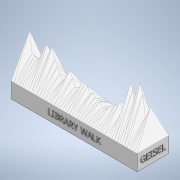
# Autodesk Inventor part: sub_base_fourier
Saved by Autodesk Inventor 2020.1 (Build 241239000, 239)
## iProperties
Created: 2019-10-01
Part Number: sub_base_fourier
Material: Generic
Document SubType Name: Modeling
Designer: Babynado
Density: 1 g/cm^3
Appearance: Default
Author: Babynado
Autodesk Inventor part; units mm, degrees
(part 1 of 3)
ref_plane "YZ Plane" through (0, 0, 0) normal (1, 0, 0) x (0, 1, 0)
ref_plane "XZ Plane" through (0, 0, 0) normal (0, 1, 0) x (-1, 0, 0)
ref_plane "XY Plane" through (0, 0, 0) normal (0, 0, 1) x (1, 0, 0)
sketch "Sketch1" plane through (0, 0, 0) normal (0, 1, 0) x (-1, 0, 0)
  line L0 (0, 0) -> (0, 50.8) projected
  line L1 (0, 50.8) -> (-203.2, 50.8) projected
  line L2 (-203.2, 0) -> (0, 0) projected
  line L3 (-203.2, 50.8) -> (-203.2, 0) projected
extrude "Extrusion1" add sketch "Sketch1" against normal blind 25.4
sketch "Sketch2" plane through (0, 0, 50.8) normal (0, 0, 1) x (1, 0, 0)
  line L0 (0, 0) -> (203.2, 0) projected
  line L1 (0, 0) -> (203.2, 0) projected
  line L2 (0, 0) -> (0, -25.4) projected
  line L3 (203.2, -25.4) -> (0, -25.4) projected
  line L4 (203.2, 0) -> (203.2, -25.4) projected
  line L5 (50.8, -8.636) -> (152.4, -8.636) construction
  line L6 (152.4, -8.636) -> (152.4, -16.764) construction
  line L7 (152.4, -16.764) -> (50.8, -16.764) construction
  line L8 (50.8, -16.764) -> (50.8, -8.636) construction
  line L9 (65.2204, -17.272) -> (59.9222, -17.272)
  line L10 (59.9222, -17.272) -> (59.9222, -8.128)
  line L11 (59.9222, -8.128) -> (61.1374, -8.128)
  line L12 (61.1374, -8.128) -> (61.1374, -16.1901)
  line L13 (61.1374, -16.1901) -> (65.2204, -16.1901)
  line L14 (65.2204, -16.1901) -> (65.2204, -17.272)
  line L15 (69.3626, -17.272) -> (65.8206, -17.272)
  line L16 (65.8206, -17.272) -> (65.8206, -16.3383)
  line L17 (65.8206, -16.3383) -> (66.984, -16.3383)
  line L18 (66.984, -16.3383) -> (66.984, -9.0617)
  line L19 (66.984, -9.0617) -> (65.8206, -9.0617)
  line L20 (65.8206, -9.0617) -> (65.8206, -8.128)
  line L21 (65.8206, -8.128) -> (69.3626, -8.128)
  line L22 (69.3626, -8.128) -> (69.3626, -9.0617)
  line L23 (69.3626, -9.0617) -> (68.1992, -9.0617)
  line L24 (68.1992, -9.0617) -> (68.1992, -16.3383)
  line L25 (68.1992, -16.3383) -> (69.3626, -16.3383)
  line L26 (69.3626, -16.3383) -> (69.3626, -17.272)
  spline S0 degree 2 poles (77.069, -14.4636) (77.069, -15.1453) (76.5503, -16.1901) (76.1205, -16.531) knots 0 0 0 1 2 2 2
  spline S1 degree 2 poles (76.1205, -16.531) (75.6018, -16.9311) (74.4236, -17.272) (73.49, -17.272) knots 0 0 0 1 2 2 2
  line L27 (73.49, -17.272) -> (70.8668, -17.272)
  line L28 (70.8668, -17.272) -> (70.8668, -8.128)
  line L29 (70.8668, -8.128) -> (73.2899, -8.128)
  spline S2 degree 2 poles (73.2899, -8.128) (74.268, -8.128) (75.2462, -8.254) (75.6908, -8.4985) knots 0 0 0 1 2 2 2
  spline S3 degree 2 poles (75.6908, -8.4985) (76.1872, -8.7579) (76.6392, -9.61) (76.6392, -10.188) knots 0 0 0 1 2 2 2
  spline S4 degree 2 poles (76.6392, -10.188) (76.6392, -10.8327) (75.9575, -11.8553) (75.3573, -12.1442) knots 0 0 0 1 2 2 2
  line L30 (75.3573, -12.1442) -> (75.3573, -12.1887)
  spline S5 degree 2 poles (75.3573, -12.1887) (76.1724, -12.411) (77.069, -13.5892) (77.069, -14.4636) knots 0 0 0 1 2 2 2
  spline S6 degree 2 poles (75.8019, -14.5155) (75.8019, -13.9968) (75.5055, -13.3299) (75.0609, -13.0927) knots 0 0 0 1 2 2 2
  spline S7 degree 2 poles (75.0609, -13.0927) (74.7719, -12.9445) (74.0902, -12.8556) (73.4603, -12.8556) knots 0 0 0 1 2 2 2
  line L31 (73.4603, -12.8556) -> (72.0821, -12.8556)
  line L32 (72.0821, -12.8556) -> (72.0821, -16.2346)
  line L33 (72.0821, -16.2346) -> (73.0676, -16.2346)
  spline S8 degree 2 poles (73.0676, -16.2346) (73.8679, -16.2346) (74.7867, -16.0864) (75.1424, -15.8493) knots 0 0 0 1 2 2 2
  spline S9 degree 2 poles (75.1424, -15.8493) (75.4833, -15.6047) (75.8019, -14.9971) (75.8019, -14.5155) knots 0 0 0 1 2 2 2
  spline S10 degree 2 poles (75.3721, -10.3584) (75.3721, -10.0324) (75.1498, -9.5433) (74.9053, -9.4025) knots 0 0 0 1 2 2 2
  spline S11 degree 2 poles (74.9053, -9.4025) (74.6089, -9.2395) (73.8901, -9.1654) (73.2454, -9.1654) knots 0 0 0 1 2 2 2
  line L34 (73.2454, -9.1654) -> (72.0821, -9.1654)
  line L35 (72.0821, -9.1654) -> (72.0821, -11.8404)
  line L36 (72.0821, -11.8404) -> (73.4603, -11.8404)
  spline S12 degree 2 poles (73.4603, -11.8404) (74.0309, -11.8404) (74.5718, -11.7219) (74.8608, -11.5366) knots 0 0 0 1 2 2 2
  spline S13 degree 2 poles (74.8608, -11.5366) (75.1424, -11.3588) (75.3721, -10.7882) (75.3721, -10.3584) knots 0 0 0 1 2 2 2
  line L37 (85.3535, -17.272) -> (83.7751, -17.272)
  line L38 (83.7751, -17.272) -> (80.8852, -13.6337)
  line L39 (80.8852, -13.6337) -> (79.4921, -13.6337)
  line L40 (79.4921, -13.6337) -> (79.4921, -17.272)
  line L41 (79.4921, -17.272) -> (78.2769, -17.272)
  line L42 (78.2769, -17.272) -> (78.2769, -8.128)
  line L43 (78.2769, -8.128) -> (80.6333, -8.128)
  spline S14 degree 2 poles (80.6333, -8.128) (81.4187, -8.128) (82.4784, -8.2984) (82.96, -8.6097) knots 0 0 0 1 2 2 2
  spline S15 degree 2 poles (82.96, -8.6097) (83.4417, -8.9209) (83.9974, -9.8916) (83.9974, -10.6104) knots 0 0 0 1 2 2 2
  spline S16 degree 2 poles (83.9974, -10.6104) (83.9974, -11.6107) (82.9748, -12.9668) (82.1005, -13.2928) knots 0 0 0 1 2 2 2
  line L44 (82.1005, -13.2928) -> (85.3535, -17.272)
  spline S17 degree 2 poles (82.7303, -10.7067) (82.7303, -10.3066) (82.4487, -9.6915) (82.1523, -9.4914) knots 0 0 0 1 2 2 2
  spline S18 degree 2 poles (82.1523, -9.4914) (81.893, -9.321) (81.2038, -9.1802) (80.7, -9.1802) knots 0 0 0 1 2 2 2
  line L45 (80.7, -9.1802) -> (79.4921, -9.1802)
  line L46 (79.4921, -9.1802) -> (79.4921, -12.6185)
  line L47 (79.4921, -12.6185) -> (80.5592, -12.6185)
  spline S19 degree 2 poles (80.5592, -12.6185) (81.0853, -12.6185) (81.9226, -12.4332) (82.2116, -12.1442) knots 0 0 0 1 2 2 2
  spline S20 degree 2 poles (82.2116, -12.1442) (82.4784, -11.8923) (82.7303, -11.1809) (82.7303, -10.7067) knots 0 0 0 1 2 2 2
  line L48 (85.0941, -17.272) -> (88.1767, -8.128)
  line L49 (88.1767, -8.128) -> (89.6735, -8.128)
  line L50 (89.6735, -8.128) -> (92.7561, -17.272)
  line L51 (92.7561, -17.272) -> (91.4742, -17.272)
  line L52 (91.4742, -17.272) -> (90.6442, -14.7155)
  line L53 (90.6442, -14.7155) -> (87.1541, -14.7155)
  line L54 (87.1541, -14.7155) -> (86.3242, -17.272)
  line L55 (86.3242, -17.272) -> (85.0941, -17.272)
  line L56 (90.3108, -13.6781) -> (88.8955, -9.3729)
  line L57 (88.8955, -9.3729) -> (87.4876, -13.6781)
  line L58 (87.4876, -13.6781) -> (90.3108, -13.6781)
  line L59 (100.6997, -17.272) -> (99.1213, -17.272)
  line L60 (99.1213, -17.272) -> (96.2314, -13.6337)
  line L61 (96.2314, -13.6337) -> (94.8383, -13.6337)
  line L62 (94.8383, -13.6337) -> (94.8383, -17.272)
  line L63 (94.8383, -17.272) -> (93.6231, -17.272)
  line L64 (93.6231, -17.272) -> (93.6231, -8.128)
  line L65 (93.6231, -8.128) -> (95.9795, -8.128)
  spline S21 degree 2 poles (95.9795, -8.128) (96.7649, -8.128) (97.8246, -8.2984) (98.3062, -8.6097) knots 0 0 0 1 2 2 2
  spline S22 degree 2 poles (98.3062, -8.6097) (98.7879, -8.9209) (99.3436, -9.8916) (99.3436, -10.6104) knots 0 0 0 1 2 2 2
  spline S23 degree 2 poles (99.3436, -10.6104) (99.3436, -11.6107) (98.3211, -12.9668) (97.4467, -13.2928) knots 0 0 0 1 2 2 2
  line L66 (97.4467, -13.2928) -> (100.6997, -17.272)
  spline S24 degree 2 poles (98.0765, -10.7067) (98.0765, -10.3066) (97.7949, -9.6915) (97.4985, -9.4914) knots 0 0 0 1 2 2 2
  spline S25 degree 2 poles (97.4985, -9.4914) (97.2392, -9.321) (96.55, -9.1802) (96.0462, -9.1802) knots 0 0 0 1 2 2 2
  line L67 (96.0462, -9.1802) -> (94.8383, -9.1802)
  line L68 (94.8383, -9.1802) -> (94.8383, -12.6185)
  line L69 (94.8383, -12.6185) -> (95.9054, -12.6185)
  spline S26 degree 2 poles (95.9054, -12.6185) (96.4315, -12.6185) (97.2688, -12.4332) (97.5578, -12.1442) knots 0 0 0 1 2 2 2
  spline S27 degree 2 poles (97.5578, -12.1442) (97.8246, -11.8923) (98.0765, -11.1809) (98.0765, -10.7067) knots 0 0 0 1 2 2 2
  line L70 (107.8281, -8.128) -> (104.7382, -13.2261)
  line L71 (104.7382, -13.2261) -> (104.7382, -17.272)
  line L72 (104.7382, -17.272) -> (103.5229, -17.272)
  line L73 (103.5229, -17.272) -> (103.5229, -13.3521)
  line L74 (103.5229, -13.3521) -> (100.4329, -8.128)
  line L75 (100.4329, -8.128) -> (101.7815, -8.128)
  line L76 (101.7815, -8.128) -> (104.1379, -12.1517)
  line L77 (104.1379, -12.1517) -> (106.5388, -8.128)
  line L78 (106.5388, -8.128) -> (107.8281, -8.128)
  line L79 (122.8483, -8.128) -> (120.5512, -17.272)
  line L80 (120.5512, -17.272) -> (119.1877, -17.272)
  line L81 (119.1877, -17.272) -> (117.3278, -9.6841)
  line L82 (117.3278, -9.6841) -> (115.5198, -17.272)
  line L83 (115.5198, -17.272) -> (114.1711, -17.272)
  line L84 (114.1711, -17.272) -> (111.837, -8.128)
  line L85 (111.837, -8.128) -> (113.0893, -8.128)
  line L86 (113.0893, -8.128) -> (114.927, -15.7085)
  line L87 (114.927, -15.7085) -> (116.7498, -8.128)
  line L88 (116.7498, -8.128) -> (117.9873, -8.128)
  line L89 (117.9873, -8.128) -> (119.825, -15.7974)
  line L90 (119.825, -15.7974) -> (121.6553, -8.128)
  line L91 (121.6553, -8.128) -> (122.8483, -8.128)
  line L92 (122.9521, -17.272) -> (126.0346, -8.128)
  line L93 (126.0346, -8.128) -> (127.5315, -8.128)
  line L94 (127.5315, -8.128) -> (130.614, -17.272)
  line L95 (130.614, -17.272) -> (129.3321, -17.272)
  line L96 (129.3321, -17.272) -> (128.5022, -14.7155)
  line L97 (128.5022, -14.7155) -> (125.012, -14.7155)
  line L98 (125.012, -14.7155) -> (124.1821, -17.272)
  line L99 (124.1821, -17.272) -> (122.9521, -17.272)
  line L100 (128.1687, -13.6781) -> (126.7534, -9.3729)
  line L101 (126.7534, -9.3729) -> (125.3455, -13.6781)
  line L102 (125.3455, -13.6781) -> (128.1687, -13.6781)
  line L103 (136.7792, -17.272) -> (131.481, -17.272)
  line L104 (131.481, -17.272) -> (131.481, -8.128)
  line L105 (131.481, -8.128) -> (132.6963, -8.128)
  line L106 (132.6963, -8.128) -> (132.6963, -16.1901)
  line L107 (132.6963, -16.1901) -> (136.7792, -16.1901)
  line L108 (136.7792, -16.1901) -> (136.7792, -17.272)
  line L109 (144.4041, -17.272) -> (142.8258, -17.272)
  line L110 (142.8258, -17.272) -> (139.4839, -13.0186)
  line L111 (139.4839, -13.0186) -> (138.9503, -13.6188)
  line L112 (138.9503, -13.6188) -> (138.9503, -17.272)
  line L113 (138.9503, -17.272) -> (137.7351, -17.272)
  line L114 (137.7351, -17.272) -> (137.7351, -8.128)
  line L115 (137.7351, -8.128) -> (138.9503, -8.128)
  line L116 (138.9503, -8.128) -> (138.9503, -12.3295)
  line L117 (138.9503, -12.3295) -> (142.6998, -8.128)
  line L118 (142.6998, -8.128) -> (144.1818, -8.128)
  line L119 (144.1818, -8.128) -> (140.3953, -12.2109)
  line L120 (140.3953, -12.2109) -> (144.4041, -17.272)
  dimension "d31" = 76.2
  dimension "d2" = 203.2
  dimension "d3" = 25.4
  dimension "d4" = 101.6
  dimension "d5" = 8.128
  dimension "d6" = 8.636
  dimension "d7" = 50.8
  constraints: 2 other
  measures "d2" distance of L0.start L0.end
  measures "d3" distance of L1.start L2.end
  measures "d4" distance of L5.start L5.end
  measures "d5" distance of L7.end L5.start
  measures "d6" distance between parallel lines of L0 L5
  measures "d7" distance between parallel lines of L2 L8
extrude "Extrusion2" cut sketch "Sketch2" against normal blind 5.08 contours L9 L10 L11 L12 L13 L14 | L15 L16 L17 L18 L19 L20 L21 L22 L23 L24 L25 L26 | S0 S1 L27 L28 L29 S2 S3 S4 L30 S5 | L37 L48 L44 | L44 L48 L49 L50 L51 L52 L53 L54 L55 | L37 L38 L39 L40 L41 L42 L43 S14 S15 S16 L44 L48 | L59 L60 L61 L62 L63 L64 L65 S21 S22 S23 L66 | L70 L71 L72 L73 L74 L75 L76 L77 L78 | L79 L80 L81 L82 L83 L84 L85 L86 L87 L88 L89 L90 L91 | L92 L93 L94 L95 L96 L97 L98 L99 | L103 L104 L105 L106 L107 L108 | L109 L110 L111 L112 L113 L114 L115 L116 L117 L118 L119 L120
sketch "Sketch3" plane through (203.2, 0, 50.8) normal (1, 0, 0) x (0, 0, -1)
  line L0 (0, 0) -> (50.8, 0) projected
  line L1 (0, 0) -> (0, -25.4) projected
  line L2 (50.8, -25.4) -> (0, -25.4) projected
  line L3 (50.8, 0) -> (50.8, -25.4) projected
  line L4 (6.35, -5.08) -> (44.45, -5.08) construction
  line L5 (44.45, -5.08) -> (44.45, -20.32) construction
  line L6 (44.45, -20.32) -> (6.35, -20.32) construction
  line L7 (6.35, -20.32) -> (6.35, -5.08) construction
  spline S0 degree 2 poles (9.9315, -17.4424) (8.9608, -17.4424) (7.3528, -16.8496) (6.7748, -16.2494) knots 0 0 0 1 2 2 2
  spline S1 degree 2 poles (6.7748, -16.2494) (6.1969, -15.6418) (5.5818, -13.8486) (5.5818, -12.6852) knots 0 0 0 1 2 2 2
  spline S2 degree 2 poles (5.5818, -12.6852) (5.5818, -11.5811) (6.2043, -9.8323) (6.7823, -9.2099) knots 0 0 0 1 2 2 2
  spline S3 degree 2 poles (6.7823, -9.2099) (7.338, -8.6097) (8.9682, -7.9576) (9.9389, -7.9576) knots 0 0 0 1 2 2 2
  spline S4 degree 2 poles (9.9389, -7.9576) (10.4058, -7.9576) (11.2505, -8.0909) (11.6358, -8.2095) knots 0 0 0 1 2 2 2
  spline S5 degree 2 poles (11.6358, -8.2095) (11.9471, -8.2984) (12.7029, -8.6245) (12.9326, -8.743) knots 0 0 0 1 2 2 2
  line L8 (12.9326, -8.743) -> (12.9326, -10.2102)
  line L9 (12.9326, -10.2102) -> (12.8289, -10.2102)
  spline S6 degree 2 poles (12.8289, -10.2102) (12.5991, -10.0102) (12.1175, -9.6471) (11.6729, -9.4396) knots 0 0 0 1 2 2 2
  spline S7 degree 2 poles (11.6729, -9.4396) (11.3024, -9.2543) (10.3465, -9.0098) (9.7981, -9.0098) knots 0 0 0 1 2 2 2
  spline S8 degree 2 poles (9.7981, -9.0098) (8.4792, -9.0098) (6.8489, -10.9957) (6.8489, -12.6481) knots 0 0 0 1 2 2 2
  spline S9 degree 2 poles (6.8489, -12.6481) (6.8489, -13.567) (7.2787, -14.9452) (7.6863, -15.4195) knots 0 0 0 1 2 2 2
  spline S10 degree 2 poles (7.6863, -15.4195) (8.079, -15.8937) (9.1905, -16.3902) (9.8871, -16.3902) knots 0 0 0 1 2 2 2
  spline S11 degree 2 poles (9.8871, -16.3902) (10.3984, -16.3902) (11.4209, -16.242) (11.7692, -16.0938) knots 0 0 0 1 2 2 2
  line L10 (11.7692, -16.0938) -> (11.7692, -13.73)
  line L11 (11.7692, -13.73) -> (9.6499, -13.73)
  line L12 (9.6499, -13.73) -> (9.6499, -12.6629)
  line L13 (9.6499, -12.6629) -> (12.9696, -12.6629)
  line L14 (12.9696, -12.6629) -> (12.9696, -16.657)
  spline S12 degree 2 poles (12.9696, -16.657) (12.7399, -16.7607) (11.9545, -17.0793) (11.621, -17.1757) knots 0 0 0 1 2 2 2
  spline S13 degree 2 poles (11.621, -17.1757) (11.169, -17.3091) (10.4428, -17.4424) (9.9315, -17.4424) knots 0 0 0 1 2 2 2
  line L15 (14.4961, -17.2646) -> (14.4961, -8.1206)
  line L16 (14.4961, -8.1206) -> (20.2167, -8.1206)
  line L17 (20.2167, -8.1206) -> (20.2167, -9.2025)
  line L18 (20.2167, -9.2025) -> (15.7114, -9.2025)
  line L19 (15.7114, -9.2025) -> (15.7114, -11.7071)
  line L20 (15.7114, -11.7071) -> (19.9129, -11.7071)
  line L21 (19.9129, -11.7071) -> (19.9129, -12.7889)
  line L22 (19.9129, -12.7889) -> (15.7114, -12.7889)
  line L23 (15.7114, -12.7889) -> (15.7114, -16.1827)
  line L24 (15.7114, -16.1827) -> (20.2167, -16.1827)
  line L25 (20.2167, -16.1827) -> (20.2167, -17.2646)
  line L26 (20.2167, -17.2646) -> (14.4961, -17.2646)
  line L27 (24.7368, -17.2646) -> (21.1948, -17.2646)
  line L28 (21.1948, -17.2646) -> (21.1948, -16.3309)
  line L29 (21.1948, -16.3309) -> (22.3582, -16.3309)
  line L30 (22.3582, -16.3309) -> (22.3582, -9.0543)
  line L31 (22.3582, -9.0543) -> (21.1948, -9.0543)
  line L32 (21.1948, -9.0543) -> (21.1948, -8.1206)
  line L33 (21.1948, -8.1206) -> (24.7368, -8.1206)
  line L34 (24.7368, -8.1206) -> (24.7368, -9.0543)
  line L35 (24.7368, -9.0543) -> (23.5734, -9.0543)
  line L36 (23.5734, -9.0543) -> (23.5734, -16.3309)
  line L37 (23.5734, -16.3309) -> (24.7368, -16.3309)
  line L38 (24.7368, -16.3309) -> (24.7368, -17.2646)
  spline S14 degree 2 poles (28.7901, -17.4276) (27.7972, -17.4276) (26.4041, -17.0126) (25.789, -16.7162) knots 0 0 0 1 2 2 2
  line L39 (25.789, -16.7162) -> (25.789, -15.1898)
  line L40 (25.789, -15.1898) -> (25.8779, -15.1898)
  spline S15 degree 2 poles (25.8779, -15.1898) (26.4782, -15.7529) (27.9972, -16.3754) (28.7012, -16.3754) knots 0 0 0 1 2 2 2
  spline S16 degree 2 poles (28.7012, -16.3754) (29.7089, -16.3754) (30.7389, -15.538) (30.7389, -14.8489) knots 0 0 0 1 2 2 2
  spline S17 degree 2 poles (30.7389, -14.8489) (30.7389, -14.3006) (30.198, -13.6188) (29.6126, -13.4484) knots 0 0 0 1 2 2 2
  spline S18 degree 2 poles (29.6126, -13.4484) (29.1902, -13.3299) (28.4863, -13.1668) (27.9602, -13.0335) knots 0 0 0 1 2 2 2
  spline S19 degree 2 poles (27.9602, -13.0335) (27.4859, -12.9075) (26.7375, -12.5296) (26.4485, -12.2258) knots 0 0 0 1 2 2 2
  spline S20 degree 2 poles (26.4485, -12.2258) (26.1669, -11.9219) (25.8557, -11.1068) (25.8557, -10.5733) knots 0 0 0 1 2 2 2
  spline S21 degree 2 poles (25.8557, -10.5733) (25.8557, -9.4618) (27.5897, -7.9576) (28.9309, -7.9576) knots 0 0 0 1 2 2 2
  spline S22 degree 2 poles (28.9309, -7.9576) (29.7015, -7.9576) (31.065, -8.2614) (31.6504, -8.5504) knots 0 0 0 1 2 2 2
  line L41 (31.6504, -8.5504) -> (31.6504, -10.0027)
  line L42 (31.6504, -10.0027) -> (31.5615, -10.0027)
  spline S23 degree 2 poles (31.5615, -10.0027) (31.1243, -9.6026) (29.7608, -9.0098) (29.0124, -9.0098) knots 0 0 0 1 2 2 2
  spline S24 degree 2 poles (29.0124, -9.0098) (28.1677, -9.0098) (27.1228, -9.8027) (27.1228, -10.4473) knots 0 0 0 1 2 2 2
  spline S25 degree 2 poles (27.1228, -10.4473) (27.1228, -11.0253) (27.7379, -11.7145) (28.3159, -11.8701) knots 0 0 0 1 2 2 2
  spline S26 degree 2 poles (28.3159, -11.8701) (28.7012, -11.9738) (29.8201, -12.2406) (30.1906, -12.3517) knots 0 0 0 1 2 2 2
  spline S27 degree 2 poles (30.1906, -12.3517) (31.1317, -12.6407) (32.0061, -13.8041) (32.0061, -14.6563) knots 0 0 0 1 2 2 2
  spline S28 degree 2 poles (32.0061, -14.6563) (32.0061, -15.1972) (31.5689, -16.2346) (31.1761, -16.5977) knots 0 0 0 1 2 2 2
  spline S29 degree 2 poles (31.1761, -16.5977) (30.7389, -16.9978) (29.6274, -17.4276) (28.7901, -17.4276) knots 0 0 0 1 2 2 2
  line L43 (33.2435, -17.2646) -> (33.2435, -8.1206)
  line L44 (33.2435, -8.1206) -> (38.9641, -8.1206)
  line L45 (38.9641, -8.1206) -> (38.9641, -9.2025)
  line L46 (38.9641, -9.2025) -> (34.4588, -9.2025)
  line L47 (34.4588, -9.2025) -> (34.4588, -11.7071)
  line L48 (34.4588, -11.7071) -> (38.6603, -11.7071)
  line L49 (38.6603, -11.7071) -> (38.6603, -12.7889)
  line L50 (38.6603, -12.7889) -> (34.4588, -12.7889)
  line L51 (34.4588, -12.7889) -> (34.4588, -16.1827)
  line L52 (34.4588, -16.1827) -> (38.9641, -16.1827)
  line L53 (38.9641, -16.1827) -> (38.9641, -17.2646)
  line L54 (38.9641, -17.2646) -> (33.2435, -17.2646)
  line L55 (45.5961, -17.2646) -> (40.2979, -17.2646)
  line L56 (40.2979, -17.2646) -> (40.2979, -8.1206)
  line L57 (40.2979, -8.1206) -> (41.5131, -8.1206)
  line L58 (41.5131, -8.1206) -> (41.5131, -16.1827)
  line L59 (41.5131, -16.1827) -> (45.5961, -16.1827)
  line L60 (45.5961, -16.1827) -> (45.5961, -17.2646)
  dimension "d10" = 50.8
  dimension "d11" = 25.4
  dimension "d12" = 38.1
  dimension "d13" = 15.24
  dimension "d14" = 6.35
  dimension "d15" = 5.08
  constraints: 2 other
  measures "d10" distance of L0.start L0.end
  measures "d11" distance of L0.start L1.end
  measures "d12" distance of L4.start L4.end
  measures "d13" distance of L6.end L4.start
  measures "d14" distance between parallel lines of L1 L7
  measures "d15" distance between parallel lines of L2 L6
extrude "Extrusion3" cut sketch "Sketch3" against normal blind 5.08 contours S0 S1 S2 S3 S4 S5 L8 L9 S6 S7 S8 S9 S10 S11 L10 L11 L12 L13 L14 S12 S13 | L15 L16 L17 L18 L19 L20 L21 L22 L23 L24 L25 L26 | L27 L28 L29 L30 L31 L32 L33 L34 L35 L36 L37 L38 | S14 L39 L40 S15 S16 S17 S18 S19 S20 S21 S22 L41 L42 S23 S24 S25 S26 S27 S28 S29 | L43 L44 L45 L46 L47 L48 L49 L50 L51 L52 L53 L54 | L55 L56 L57 L58 L59 L60
sketch "Sketch4" plane through (203.2, 0, 0) normal (0, 0, -1) x (-1, 0, 0)
  line L0 (0, 0) -> (203.2, 0) projected
  line L1 (0, 0) -> (0, -25.4) projected
  line L2 (203.2, -25.4) -> (0, -25.4) projected
  line L3 (203.2, 0) -> (203.2, -25.4) projected
  line L4 (0, -7.62) -> (203.2, -7.62) construction
  line L5 (203.2, -7.62) -> (203.2, -17.78) construction
  line L6 (203.2, -17.78) -> (0, -17.78) construction
  line L7 (0, -17.78) -> (0, -7.62) construction
  spline S0 degree 2 poles (11.9829, -17.435) (10.9899, -17.435) (9.5968, -17.0201) (8.9818, -16.7237) knots 0 0 0 1 2 2 2
  line L8 (8.9818, -16.7237) -> (8.9818, -15.1972)
  line L9 (8.9818, -15.1972) -> (9.0707, -15.1972)
  spline S1 degree 2 poles (9.0707, -15.1972) (9.6709, -15.7604) (11.19, -16.3828) (11.894, -16.3828) knots 0 0 0 1 2 2 2
  spline S2 degree 2 poles (11.894, -16.3828) (12.9017, -16.3828) (13.9317, -15.5455) (13.9317, -14.8563) knots 0 0 0 1 2 2 2
  spline S3 degree 2 poles (13.9317, -14.8563) (13.9317, -14.308) (13.3908, -13.6263) (12.8054, -13.4558) knots 0 0 0 1 2 2 2
  spline S4 degree 2 poles (12.8054, -13.4558) (12.383, -13.3373) (11.6791, -13.1742) (11.153, -13.0409) knots 0 0 0 1 2 2 2
  spline S5 degree 2 poles (11.153, -13.0409) (10.6787, -12.9149) (9.9303, -12.537) (9.6413, -12.2332) knots 0 0 0 1 2 2 2
  spline S6 degree 2 poles (9.6413, -12.2332) (9.3597, -11.9294) (9.0485, -11.1142) (9.0485, -10.5807) knots 0 0 0 1 2 2 2
  spline S7 degree 2 poles (9.0485, -10.5807) (9.0485, -9.4692) (10.7825, -7.965) (12.1237, -7.965) knots 0 0 0 1 2 2 2
  spline S8 degree 2 poles (12.1237, -7.965) (12.8943, -7.965) (14.2578, -8.2688) (14.8432, -8.5578) knots 0 0 0 1 2 2 2
  line L10 (14.8432, -8.5578) -> (14.8432, -10.0102)
  line L11 (14.8432, -10.0102) -> (14.7542, -10.0102)
  spline S9 degree 2 poles (14.7542, -10.0102) (14.317, -9.61) (12.9536, -9.0172) (12.2052, -9.0172) knots 0 0 0 1 2 2 2
  spline S10 degree 2 poles (12.2052, -9.0172) (11.3604, -9.0172) (10.3156, -9.8101) (10.3156, -10.4548) knots 0 0 0 1 2 2 2
  spline S11 degree 2 poles (10.3156, -10.4548) (10.3156, -11.0327) (10.9307, -11.7219) (11.5086, -11.8775) knots 0 0 0 1 2 2 2
  spline S12 degree 2 poles (11.5086, -11.8775) (11.894, -11.9812) (13.0129, -12.248) (13.3834, -12.3591) knots 0 0 0 1 2 2 2
  spline S13 degree 2 poles (13.3834, -12.3591) (14.3245, -12.6481) (15.1988, -13.8115) (15.1988, -14.6637) knots 0 0 0 1 2 2 2
  spline S14 degree 2 poles (15.1988, -14.6637) (15.1988, -15.2046) (14.7616, -16.242) (14.3689, -16.6051) knots 0 0 0 1 2 2 2
  spline S15 degree 2 poles (14.3689, -16.6051) (13.9317, -17.0052) (12.8202, -17.435) (11.9829, -17.435) knots 0 0 0 1 2 2 2
  spline S16 degree 2 poles (19.6301, -17.4647) (18.8224, -17.4647) (17.6219, -17.0423) (17.1996, -16.6199) knots 0 0 0 1 2 2 2
  spline S17 degree 2 poles (17.1996, -16.6199) (16.7179, -16.1457) (16.3252, -14.8119) (16.3252, -13.8337) knots 0 0 0 1 2 2 2
  line L12 (16.3252, -13.8337) -> (16.3252, -8.128)
  line L13 (16.3252, -8.128) -> (17.5404, -8.128)
  line L14 (17.5404, -8.128) -> (17.5404, -13.8337)
  spline S18 degree 2 poles (17.5404, -13.8337) (17.5404, -14.471) (17.7034, -15.3306) (17.9331, -15.6788) knots 0 0 0 1 2 2 2
  spline S19 degree 2 poles (17.9331, -15.6788) (18.1777, -16.0493) (19.0224, -16.4273) (19.6301, -16.4273) knots 0 0 0 1 2 2 2
  spline S20 degree 2 poles (19.6301, -16.4273) (20.2006, -16.4273) (21.0898, -16.0493) (21.3344, -15.6788) knots 0 0 0 1 2 2 2
  spline S21 degree 2 poles (21.3344, -15.6788) (21.5641, -15.3306) (21.7271, -14.4784) (21.7271, -13.8634) knots 0 0 0 1 2 2 2
  line L15 (21.7271, -13.8634) -> (21.7271, -8.128)
  line L16 (21.7271, -8.128) -> (22.9423, -8.128)
  line L17 (22.9423, -8.128) -> (22.9423, -13.8337)
  spline S22 degree 2 poles (22.9423, -13.8337) (22.9423, -14.7896) (22.557, -16.1531) (22.068, -16.6199) knots 0 0 0 1 2 2 2
  spline S23 degree 2 poles (22.068, -16.6199) (21.6308, -17.0497) (20.4748, -17.4647) (19.6301, -17.4647) knots 0 0 0 1 2 2 2
  spline S24 degree 2 poles (30.8859, -14.4636) (30.8859, -15.1453) (30.3672, -16.1901) (29.9374, -16.531) knots 0 0 0 1 2 2 2
  spline S25 degree 2 poles (29.9374, -16.531) (29.4187, -16.9311) (28.2405, -17.272) (27.3069, -17.272) knots 0 0 0 1 2 2 2
  line L18 (27.3069, -17.272) -> (24.6837, -17.272)
  line L19 (24.6837, -17.272) -> (24.6837, -8.128)
  line L20 (24.6837, -8.128) -> (27.1068, -8.128)
  spline S26 degree 2 poles (27.1068, -8.128) (28.0849, -8.128) (29.063, -8.254) (29.5076, -8.4985) knots 0 0 0 1 2 2 2
  spline S27 degree 2 poles (29.5076, -8.4985) (30.0041, -8.7579) (30.4561, -9.61) (30.4561, -10.188) knots 0 0 0 1 2 2 2
  spline S28 degree 2 poles (30.4561, -10.188) (30.4561, -10.8327) (29.7744, -11.8553) (29.1742, -12.1442) knots 0 0 0 1 2 2 2
  line L21 (29.1742, -12.1442) -> (29.1742, -12.1887)
  spline S29 degree 2 poles (29.1742, -12.1887) (29.9893, -12.411) (30.8859, -13.5892) (30.8859, -14.4636) knots 0 0 0 1 2 2 2
  spline S30 degree 2 poles (29.6188, -14.5155) (29.6188, -13.9968) (29.3224, -13.3299) (28.8778, -13.0927) knots 0 0 0 1 2 2 2
  spline S31 degree 2 poles (28.8778, -13.0927) (28.5888, -12.9445) (27.9071, -12.8556) (27.2772, -12.8556) knots 0 0 0 1 2 2 2
  line L22 (27.2772, -12.8556) -> (25.899, -12.8556)
  line L23 (25.899, -12.8556) -> (25.899, -16.2346)
  line L24 (25.899, -16.2346) -> (26.8845, -16.2346)
  spline S32 degree 2 poles (26.8845, -16.2346) (27.6848, -16.2346) (28.6036, -16.0864) (28.9593, -15.8493) knots 0 0 0 1 2 2 2
  spline S33 degree 2 poles (28.9593, -15.8493) (29.3002, -15.6047) (29.6188, -14.9971) (29.6188, -14.5155) knots 0 0 0 1 2 2 2
  spline S34 degree 2 poles (29.189, -10.3584) (29.189, -10.0324) (28.9667, -9.5433) (28.7222, -9.4025) knots 0 0 0 1 2 2 2
  spline S35 degree 2 poles (28.7222, -9.4025) (28.4258, -9.2395) (27.707, -9.1654) (27.0623, -9.1654) knots 0 0 0 1 2 2 2
  line L25 (27.0623, -9.1654) -> (25.899, -9.1654)
  line L26 (25.899, -9.1654) -> (25.899, -11.8404)
  line L27 (25.899, -11.8404) -> (27.2772, -11.8404)
  spline S36 degree 2 poles (27.2772, -11.8404) (27.8478, -11.8404) (28.3887, -11.7219) (28.6777, -11.5366) knots 0 0 0 1 2 2 2
  spline S37 degree 2 poles (28.6777, -11.5366) (28.9593, -11.3588) (29.189, -10.7882) (29.189, -10.3584) knots 0 0 0 1 2 2 2
  line L28 (35.1837, -13.8263) -> (31.7232, -13.8263)
  line L29 (31.7232, -13.8263) -> (31.7232, -12.7148)
  line L30 (31.7232, -12.7148) -> (35.1837, -12.7148)
  line L31 (35.1837, -12.7148) -> (35.1837, -13.8263)
  spline S38 degree 2 poles (42.8606, -14.4636) (42.8606, -15.1453) (42.3418, -16.1901) (41.9121, -16.531) knots 0 0 0 1 2 2 2
  spline S39 degree 2 poles (41.9121, -16.531) (41.3934, -16.9311) (40.2152, -17.272) (39.2815, -17.272) knots 0 0 0 1 2 2 2
  line L32 (39.2815, -17.272) -> (36.6583, -17.272)
  line L33 (36.6583, -17.272) -> (36.6583, -8.128)
  line L34 (36.6583, -8.128) -> (39.0814, -8.128)
  spline S40 degree 2 poles (39.0814, -8.128) (40.0596, -8.128) (41.0377, -8.254) (41.4823, -8.4985) knots 0 0 0 1 2 2 2
  spline S41 degree 2 poles (41.4823, -8.4985) (41.9788, -8.7579) (42.4308, -9.61) (42.4308, -10.188) knots 0 0 0 1 2 2 2
  spline S42 degree 2 poles (42.4308, -10.188) (42.4308, -10.8327) (41.749, -11.8553) (41.1488, -12.1442) knots 0 0 0 1 2 2 2
  line L35 (41.1488, -12.1442) -> (41.1488, -12.1887)
  spline S43 degree 2 poles (41.1488, -12.1887) (41.9639, -12.411) (42.8606, -13.5892) (42.8606, -14.4636) knots 0 0 0 1 2 2 2
  spline S44 degree 2 poles (41.5934, -14.5155) (41.5934, -13.9968) (41.297, -13.3299) (40.8524, -13.0927) knots 0 0 0 1 2 2 2
  spline S45 degree 2 poles (40.8524, -13.0927) (40.5634, -12.9445) (39.8817, -12.8556) (39.2519, -12.8556) knots 0 0 0 1 2 2 2
  line L36 (39.2519, -12.8556) -> (37.8736, -12.8556)
  line L37 (37.8736, -12.8556) -> (37.8736, -16.2346)
  line L38 (37.8736, -16.2346) -> (38.8591, -16.2346)
  spline S46 degree 2 poles (38.8591, -16.2346) (39.6594, -16.2346) (40.5783, -16.0864) (40.9339, -15.8493) knots 0 0 0 1 2 2 2
  spline S47 degree 2 poles (40.9339, -15.8493) (41.2748, -15.6047) (41.5934, -14.9971) (41.5934, -14.5155) knots 0 0 0 1 2 2 2
  spline S48 degree 2 poles (41.1637, -10.3584) (41.1637, -10.0324) (40.9414, -9.5433) (40.6968, -9.4025) knots 0 0 0 1 2 2 2
  spline S49 degree 2 poles (40.6968, -9.4025) (40.4004, -9.2395) (39.6816, -9.1654) (39.037, -9.1654) knots 0 0 0 1 2 2 2
  line L39 (39.037, -9.1654) -> (37.8736, -9.1654)
  line L40 (37.8736, -9.1654) -> (37.8736, -11.8404)
  line L41 (37.8736, -11.8404) -> (39.2519, -11.8404)
  spline S50 degree 2 poles (39.2519, -11.8404) (39.8224, -11.8404) (40.3634, -11.7219) (40.6524, -11.5366) knots 0 0 0 1 2 2 2
  spline S51 degree 2 poles (40.6524, -11.5366) (40.9339, -11.3588) (41.1637, -10.7882) (41.1637, -10.3584) knots 0 0 0 1 2 2 2
  line L42 (43.0829, -17.272) -> (46.1654, -8.128)
  line L43 (46.1654, -8.128) -> (47.6623, -8.128)
  line L44 (47.6623, -8.128) -> (50.7448, -17.272)
  line L45 (50.7448, -17.272) -> (49.4629, -17.272)
  line L46 (49.4629, -17.272) -> (48.633, -14.7155)
  line L47 (48.633, -14.7155) -> (45.1428, -14.7155)
  line L48 (45.1428, -14.7155) -> (44.3129, -17.272)
  line L49 (44.3129, -17.272) -> (43.0829, -17.272)
  line L50 (48.2995, -13.6781) -> (46.8842, -9.3729)
  line L51 (46.8842, -9.3729) -> (45.4763, -13.6781)
  line L52 (45.4763, -13.6781) -> (48.2995, -13.6781)
  spline S52 degree 2 poles (54.1609, -17.435) (53.1679, -17.435) (51.7748, -17.0201) (51.1598, -16.7237) knots 0 0 0 1 2 2 2
  line L53 (51.1598, -16.7237) -> (51.1598, -15.1972)
  line L54 (51.1598, -15.1972) -> (51.2487, -15.1972)
  spline S53 degree 2 poles (51.2487, -15.1972) (51.8489, -15.7604) (53.368, -16.3828) (54.072, -16.3828) knots 0 0 0 1 2 2 2
  spline S54 degree 2 poles (54.072, -16.3828) (55.0797, -16.3828) (56.1097, -15.5455) (56.1097, -14.8563) knots 0 0 0 1 2 2 2
  spline S55 degree 2 poles (56.1097, -14.8563) (56.1097, -14.308) (55.5688, -13.6263) (54.9834, -13.4558) knots 0 0 0 1 2 2 2
  spline S56 degree 2 poles (54.9834, -13.4558) (54.561, -13.3373) (53.8571, -13.1742) (53.331, -13.0409) knots 0 0 0 1 2 2 2
  spline S57 degree 2 poles (53.331, -13.0409) (52.8567, -12.9149) (52.1083, -12.537) (51.8193, -12.2332) knots 0 0 0 1 2 2 2
  spline S58 degree 2 poles (51.8193, -12.2332) (51.5377, -11.9294) (51.2265, -11.1142) (51.2265, -10.5807) knots 0 0 0 1 2 2 2
  spline S59 degree 2 poles (51.2265, -10.5807) (51.2265, -9.4692) (52.9604, -7.965) (54.3017, -7.965) knots 0 0 0 1 2 2 2
  spline S60 degree 2 poles (54.3017, -7.965) (55.0723, -7.965) (56.4358, -8.2688) (57.0212, -8.5578) knots 0 0 0 1 2 2 2
  line L55 (57.0212, -8.5578) -> (57.0212, -10.0102)
  line L56 (57.0212, -10.0102) -> (56.9322, -10.0102)
  spline S61 degree 2 poles (56.9322, -10.0102) (56.495, -9.61) (55.1316, -9.0172) (54.3832, -9.0172) knots 0 0 0 1 2 2 2
  spline S62 degree 2 poles (54.3832, -9.0172) (53.5384, -9.0172) (52.4936, -9.8101) (52.4936, -10.4548) knots 0 0 0 1 2 2 2
  spline S63 degree 2 poles (52.4936, -10.4548) (52.4936, -11.0327) (53.1086, -11.7219) (53.6866, -11.8775) knots 0 0 0 1 2 2 2
  spline S64 degree 2 poles (53.6866, -11.8775) (54.072, -11.9812) (55.1909, -12.248) (55.5614, -12.3591) knots 0 0 0 1 2 2 2
  spline S65 degree 2 poles (55.5614, -12.3591) (56.5025, -12.6481) (57.3768, -13.8115) (57.3768, -14.6637) knots 0 0 0 1 2 2 2
  spline S66 degree 2 poles (57.3768, -14.6637) (57.3768, -15.2046) (56.9396, -16.242) (56.5469, -16.6051) knots 0 0 0 1 2 2 2
  spline S67 degree 2 poles (56.5469, -16.6051) (56.1097, -17.0052) (54.9982, -17.435) (54.1609, -17.435) knots 0 0 0 1 2 2 2
  line L57 (58.6143, -17.272) -> (58.6143, -8.128)
  line L58 (58.6143, -8.128) -> (64.3349, -8.128)
  line L59 (64.3349, -8.128) -> (64.3349, -9.2099)
  line L60 (64.3349, -9.2099) -> (59.8296, -9.2099)
  line L61 (59.8296, -9.2099) -> (59.8296, -11.7145)
  line L62 (59.8296, -11.7145) -> (64.0311, -11.7145)
  line L63 (64.0311, -11.7145) -> (64.0311, -12.7963)
  line L64 (64.0311, -12.7963) -> (59.8296, -12.7963)
  line L65 (59.8296, -12.7963) -> (59.8296, -16.1901)
  line L66 (59.8296, -16.1901) -> (64.3349, -16.1901)
  line L67 (64.3349, -16.1901) -> (64.3349, -17.272)
  line L68 (64.3349, -17.272) -> (58.6143, -17.272)
  line L69 (75.0646, -9.2099) -> (70.8113, -9.2099)
  line L70 (70.8113, -9.2099) -> (70.8113, -11.7886)
  line L71 (70.8113, -11.7886) -> (74.8868, -11.7886)
  line L72 (74.8868, -11.7886) -> (74.8868, -12.8704)
  line L73 (74.8868, -12.8704) -> (70.8113, -12.8704)
  line L74 (70.8113, -12.8704) -> (70.8113, -17.272)
  line L75 (70.8113, -17.272) -> (69.596, -17.272)
  line L76 (69.596, -17.272) -> (69.596, -8.128)
  line L77 (69.596, -8.128) -> (75.0646, -8.128)
  line L78 (75.0646, -8.128) -> (75.0646, -9.2099)
  spline S68 degree 2 poles (82.6229, -9.1728) (83.1416, -9.7804) (83.7196, -11.5589) (83.7196, -12.7) knots 0 0 0 1 2 2 2
  spline S69 degree 2 poles (83.7196, -12.7) (83.7196, -13.8115) (83.1564, -15.6121) (82.6229, -16.2198) knots 0 0 0 1 2 2 2
  spline S70 degree 2 poles (82.6229, -16.2198) (82.0597, -16.857) (80.5703, -17.4647) (79.6737, -17.4647) knots 0 0 0 1 2 2 2
  spline S71 degree 2 poles (79.6737, -17.4647) (78.7474, -17.4647) (77.2654, -16.8348) (76.7245, -16.2198) knots 0 0 0 1 2 2 2
  spline S72 degree 2 poles (76.7245, -16.2198) (76.1984, -15.6121) (75.6352, -13.8263) (75.6352, -12.7) knots 0 0 0 1 2 2 2
  spline S73 degree 2 poles (75.6352, -12.7) (75.6352, -11.5514) (76.2058, -9.8027) (76.7319, -9.1728) knots 0 0 0 1 2 2 2
  spline S74 degree 2 poles (76.7319, -9.1728) (77.2654, -8.5652) (78.7548, -7.9353) (79.6737, -7.9353) knots 0 0 0 1 2 2 2
  spline S75 degree 2 poles (79.6737, -7.9353) (80.6073, -7.9353) (82.1042, -8.5874) (82.6229, -9.1728) knots 0 0 0 1 2 2 2
  spline S76 degree 2 poles (82.4524, -12.7) (82.4524, -11.796) (82.0597, -10.3955) (81.704, -9.9361) knots 0 0 0 1 2 2 2
  spline S77 degree 2 poles (81.704, -9.9361) (81.3409, -9.4618) (80.3183, -8.9876) (79.6811, -8.9876) knots 0 0 0 1 2 2 2
  spline S78 degree 2 poles (79.6811, -8.9876) (79.0216, -8.9876) (78.0286, -9.447) (77.6507, -9.9361) knots 0 0 0 1 2 2 2
  spline S79 degree 2 poles (77.6507, -9.9361) (77.2876, -10.4029) (76.9023, -11.8108) (76.9023, -12.7) knots 0 0 0 1 2 2 2
  spline S80 degree 2 poles (76.9023, -12.7) (76.9023, -14.5006) (78.414, -16.4124) (79.6811, -16.4124) knots 0 0 0 1 2 2 2
  spline S81 degree 2 poles (79.6811, -16.4124) (80.9482, -16.4124) (82.4524, -14.5006) (82.4524, -12.7) knots 0 0 0 1 2 2 2
  spline S82 degree 2 poles (88.2471, -17.4647) (87.4394, -17.4647) (86.239, -17.0423) (85.8166, -16.6199) knots 0 0 0 1 2 2 2
  spline S83 degree 2 poles (85.8166, -16.6199) (85.335, -16.1457) (84.9422, -14.8119) (84.9422, -13.8337) knots 0 0 0 1 2 2 2
  line L79 (84.9422, -13.8337) -> (84.9422, -8.128)
  line L80 (84.9422, -8.128) -> (86.1575, -8.128)
  line L81 (86.1575, -8.128) -> (86.1575, -13.8337)
  spline S84 degree 2 poles (86.1575, -13.8337) (86.1575, -14.471) (86.3205, -15.3306) (86.5502, -15.6788) knots 0 0 0 1 2 2 2
  spline S85 degree 2 poles (86.5502, -15.6788) (86.7947, -16.0493) (87.6395, -16.4273) (88.2471, -16.4273) knots 0 0 0 1 2 2 2
  spline S86 degree 2 poles (88.2471, -16.4273) (88.8177, -16.4273) (89.7069, -16.0493) (89.9514, -15.6788) knots 0 0 0 1 2 2 2
  spline S87 degree 2 poles (89.9514, -15.6788) (90.1811, -15.3306) (90.3441, -14.4784) (90.3441, -13.8634) knots 0 0 0 1 2 2 2
  line L82 (90.3441, -13.8634) -> (90.3441, -8.128)
  line L83 (90.3441, -8.128) -> (91.5594, -8.128)
  line L84 (91.5594, -8.128) -> (91.5594, -13.8337)
  spline S88 degree 2 poles (91.5594, -13.8337) (91.5594, -14.7896) (91.1741, -16.1531) (90.685, -16.6199) knots 0 0 0 1 2 2 2
  spline S89 degree 2 poles (90.685, -16.6199) (90.2478, -17.0497) (89.0918, -17.4647) (88.2471, -17.4647) knots 0 0 0 1 2 2 2
  line L85 (100.3773, -17.272) -> (98.799, -17.272)
  line L86 (98.799, -17.272) -> (95.9091, -13.6337)
  line L87 (95.9091, -13.6337) -> (94.516, -13.6337)
  line L88 (94.516, -13.6337) -> (94.516, -17.272)
  line L89 (94.516, -17.272) -> (93.3008, -17.272)
  line L90 (93.3008, -17.272) -> (93.3008, -8.128)
  line L91 (93.3008, -8.128) -> (95.6571, -8.128)
  spline S90 degree 2 poles (95.6571, -8.128) (96.4426, -8.128) (97.5023, -8.2984) (97.9839, -8.6097) knots 0 0 0 1 2 2 2
  spline S91 degree 2 poles (97.9839, -8.6097) (98.4656, -8.9209) (99.0213, -9.8916) (99.0213, -10.6104) knots 0 0 0 1 2 2 2
  spline S92 degree 2 poles (99.0213, -10.6104) (99.0213, -11.6107) (97.9987, -12.9668) (97.1243, -13.2928) knots 0 0 0 1 2 2 2
  line L92 (97.1243, -13.2928) -> (100.3773, -17.272)
  spline S93 degree 2 poles (97.7542, -10.7067) (97.7542, -10.3066) (97.4726, -9.6915) (97.1762, -9.4914) knots 0 0 0 1 2 2 2
  spline S94 degree 2 poles (97.1762, -9.4914) (96.9169, -9.321) (96.2277, -9.1802) (95.7238, -9.1802) knots 0 0 0 1 2 2 2
  line L93 (95.7238, -9.1802) -> (94.516, -9.1802)
  line L94 (94.516, -9.1802) -> (94.516, -12.6185)
  line L95 (94.516, -12.6185) -> (95.583, -12.6185)
  spline S95 degree 2 poles (95.583, -12.6185) (96.1092, -12.6185) (96.9465, -12.4332) (97.2355, -12.1442) knots 0 0 0 1 2 2 2
  spline S96 degree 2 poles (97.2355, -12.1442) (97.5023, -11.8923) (97.7542, -11.1809) (97.7542, -10.7067) knots 0 0 0 1 2 2 2
  line L96 (104.2899, -17.272) -> (100.7479, -17.272)
  line L97 (100.7479, -17.272) -> (100.7479, -16.3383)
  line L98 (100.7479, -16.3383) -> (101.9112, -16.3383)
  line L99 (101.9112, -16.3383) -> (101.9112, -9.0617)
  line L100 (101.9112, -9.0617) -> (100.7479, -9.0617)
  line L101 (100.7479, -9.0617) -> (100.7479, -8.128)
  line L102 (100.7479, -8.128) -> (104.2899, -8.128)
  line L103 (104.2899, -8.128) -> (104.2899, -9.0617)
  line L104 (104.2899, -9.0617) -> (103.1265, -9.0617)
  line L105 (103.1265, -9.0617) -> (103.1265, -16.3383)
  line L106 (103.1265, -16.3383) -> (104.2899, -16.3383)
  line L107 (104.2899, -16.3383) -> (104.2899, -17.272)
  line L108 (105.7941, -17.272) -> (105.7941, -8.128)
  line L109 (105.7941, -8.128) -> (111.5147, -8.128)
  line L110 (111.5147, -8.128) -> (111.5147, -9.2099)
  line L111 (111.5147, -9.2099) -> (107.0093, -9.2099)
  line L112 (107.0093, -9.2099) -> (107.0093, -11.7145)
  line L113 (107.0093, -11.7145) -> (111.2108, -11.7145)
  line L114 (111.2108, -11.7145) -> (111.2108, -12.7963)
  line L115 (111.2108, -12.7963) -> (107.0093, -12.7963)
  line L116 (107.0093, -12.7963) -> (107.0093, -16.1901)
  line L117 (107.0093, -16.1901) -> (111.5147, -16.1901)
  line L118 (111.5147, -16.1901) -> (111.5147, -17.272)
  line L119 (111.5147, -17.272) -> (105.7941, -17.272)
  line L120 (119.9251, -17.272) -> (118.3467, -17.272)
  line L121 (118.3467, -17.272) -> (115.4568, -13.6337)
  line L122 (115.4568, -13.6337) -> (114.0637, -13.6337)
  line L123 (114.0637, -13.6337) -> (114.0637, -17.272)
  line L124 (114.0637, -17.272) -> (112.8485, -17.272)
  line L125 (112.8485, -17.272) -> (112.8485, -8.128)
  line L126 (112.8485, -8.128) -> (115.2049, -8.128)
  spline S97 degree 2 poles (115.2049, -8.128) (115.9903, -8.128) (117.05, -8.2984) (117.5316, -8.6097) knots 0 0 0 1 2 2 2
  spline S98 degree 2 poles (117.5316, -8.6097) (118.0133, -8.9209) (118.569, -9.8916) (118.569, -10.6104) knots 0 0 0 1 2 2 2
  spline S99 degree 2 poles (118.569, -10.6104) (118.569, -11.6107) (117.5464, -12.9668) (116.672, -13.2928) knots 0 0 0 1 2 2 2
  line L127 (116.672, -13.2928) -> (119.9251, -17.272)
  spline S100 degree 2 poles (117.3019, -10.7067) (117.3019, -10.3066) (117.0203, -9.6915) (116.7239, -9.4914) knots 0 0 0 1 2 2 2
  spline S101 degree 2 poles (116.7239, -9.4914) (116.4646, -9.321) (115.7754, -9.1802) (115.2715, -9.1802) knots 0 0 0 1 2 2 2
  line L128 (115.2715, -9.1802) -> (114.0637, -9.1802)
  line L129 (114.0637, -9.1802) -> (114.0637, -12.6185)
  line L130 (114.0637, -12.6185) -> (115.1308, -12.6185)
  spline S102 degree 2 poles (115.1308, -12.6185) (115.6569, -12.6185) (116.4942, -12.4332) (116.7832, -12.1442) knots 0 0 0 1 2 2 2
  spline S103 degree 2 poles (116.7832, -12.1442) (117.05, -11.8923) (117.3019, -11.1809) (117.3019, -10.7067) knots 0 0 0 1 2 2 2
  line L131 (126.7127, -17.272) -> (126.7127, -9.2099)
  line L132 (126.7127, -9.2099) -> (123.6449, -9.2099)
  line L133 (123.6449, -9.2099) -> (123.6449, -8.128)
  line L134 (123.6449, -8.128) -> (130.9957, -8.128)
  line L135 (130.9957, -8.128) -> (130.9957, -9.2099)
  line L136 (130.9957, -9.2099) -> (127.9279, -9.2099)
  line L137 (127.9279, -9.2099) -> (127.9279, -17.272)
  line L138 (127.9279, -17.272) -> (126.7127, -17.272)
  line L139 (138.9985, -17.272) -> (137.4202, -17.272)
  line L140 (137.4202, -17.272) -> (134.5303, -13.6337)
  line L141 (134.5303, -13.6337) -> (133.1372, -13.6337)
  line L142 (133.1372, -13.6337) -> (133.1372, -17.272)
  line L143 (133.1372, -17.272) -> (131.9219, -17.272)
  line L144 (131.9219, -17.272) -> (131.9219, -8.128)
  line L145 (131.9219, -8.128) -> (134.2783, -8.128)
  spline S104 degree 2 poles (134.2783, -8.128) (135.0638, -8.128) (136.1234, -8.2984) (136.6051, -8.6097) knots 0 0 0 1 2 2 2
  spline S105 degree 2 poles (136.6051, -8.6097) (137.0867, -8.9209) (137.6425, -9.8916) (137.6425, -10.6104) knots 0 0 0 1 2 2 2
  spline S106 degree 2 poles (137.6425, -10.6104) (137.6425, -11.6107) (136.6199, -12.9668) (135.7455, -13.2928) knots 0 0 0 1 2 2 2
  line L146 (135.7455, -13.2928) -> (138.9985, -17.272)
  spline S107 degree 2 poles (136.3754, -10.7067) (136.3754, -10.3066) (136.0938, -9.6915) (135.7974, -9.4914) knots 0 0 0 1 2 2 2
  spline S108 degree 2 poles (135.7974, -9.4914) (135.538, -9.321) (134.8489, -9.1802) (134.345, -9.1802) knots 0 0 0 1 2 2 2
  line L147 (134.345, -9.1802) -> (133.1372, -9.1802)
  line L148 (133.1372, -9.1802) -> (133.1372, -12.6185)
  line L149 (133.1372, -12.6185) -> (134.2042, -12.6185)
  spline S109 degree 2 poles (134.2042, -12.6185) (134.7303, -12.6185) (135.5677, -12.4332) (135.8567, -12.1442) knots 0 0 0 1 2 2 2
  spline S110 degree 2 poles (135.8567, -12.1442) (136.1234, -11.8923) (136.3754, -11.1809) (136.3754, -10.7067) knots 0 0 0 1 2 2 2
  line L150 (138.7392, -17.272) -> (141.8218, -8.128)
  line L151 (141.8218, -8.128) -> (143.3186, -8.128)
  line L152 (143.3186, -8.128) -> (146.4012, -17.272)
  line L153 (146.4012, -17.272) -> (145.1192, -17.272)
  line L154 (145.1192, -17.272) -> (144.2893, -14.7155)
  line L155 (144.2893, -14.7155) -> (140.7992, -14.7155)
  line L156 (140.7992, -14.7155) -> (139.9692, -17.272)
  line L157 (139.9692, -17.272) -> (138.7392, -17.272)
  line L158 (143.9558, -13.6781) -> (142.5405, -9.3729)
  line L159 (142.5405, -9.3729) -> (141.1326, -13.6781)
  line L160 (141.1326, -13.6781) -> (143.9558, -13.6781)
  line L161 (153.8112, -17.272) -> (152.4478, -17.272)
  line L162 (152.4478, -17.272) -> (148.4019, -9.3877)
  line L163 (148.4019, -9.3877) -> (148.4019, -17.272)
  line L164 (148.4019, -17.272) -> (147.2681, -17.272)
  line L165 (147.2681, -17.272) -> (147.2681, -8.128)
  line L166 (147.2681, -8.128) -> (148.9947, -8.128)
  line L167 (148.9947, -8.128) -> (152.6775, -15.3676)
  line L168 (152.6775, -15.3676) -> (152.6775, -8.128)
  line L169 (152.6775, -8.128) -> (153.8112, -8.128)
  line L170 (153.8112, -8.128) -> (153.8112, -17.272)
  spline S111 degree 2 poles (158.2128, -17.435) (157.2198, -17.435) (155.8267, -17.0201) (155.2117, -16.7237) knots 0 0 0 1 2 2 2
  line L171 (155.2117, -16.7237) -> (155.2117, -15.1972)
  line L172 (155.2117, -15.1972) -> (155.3006, -15.1972)
  spline S112 degree 2 poles (155.3006, -15.1972) (155.9008, -15.7604) (157.4199, -16.3828) (158.1239, -16.3828) knots 0 0 0 1 2 2 2
  spline S113 degree 2 poles (158.1239, -16.3828) (159.1316, -16.3828) (160.1616, -15.5455) (160.1616, -14.8563) knots 0 0 0 1 2 2 2
  spline S114 degree 2 poles (160.1616, -14.8563) (160.1616, -14.308) (159.6207, -13.6263) (159.0353, -13.4558) knots 0 0 0 1 2 2 2
  spline S115 degree 2 poles (159.0353, -13.4558) (158.6129, -13.3373) (157.909, -13.1742) (157.3829, -13.0409) knots 0 0 0 1 2 2 2
  spline S116 degree 2 poles (157.3829, -13.0409) (156.9086, -12.9149) (156.1602, -12.537) (155.8712, -12.2332) knots 0 0 0 1 2 2 2
  spline S117 degree 2 poles (155.8712, -12.2332) (155.5896, -11.9294) (155.2784, -11.1142) (155.2784, -10.5807) knots 0 0 0 1 2 2 2
  spline S118 degree 2 poles (155.2784, -10.5807) (155.2784, -9.4692) (157.0123, -7.965) (158.3536, -7.965) knots 0 0 0 1 2 2 2
  spline S119 degree 2 poles (158.3536, -7.965) (159.1242, -7.965) (160.4877, -8.2688) (161.0731, -8.5578) knots 0 0 0 1 2 2 2
  line L173 (161.0731, -8.5578) -> (161.0731, -10.0102)
  line L174 (161.0731, -10.0102) -> (160.9841, -10.0102)
  spline S120 degree 2 poles (160.9841, -10.0102) (160.5469, -9.61) (159.1835, -9.0172) (158.4351, -9.0172) knots 0 0 0 1 2 2 2
  spline S121 degree 2 poles (158.4351, -9.0172) (157.5903, -9.0172) (156.5455, -9.8101) (156.5455, -10.4548) knots 0 0 0 1 2 2 2
  spline S122 degree 2 poles (156.5455, -10.4548) (156.5455, -11.0327) (157.1606, -11.7219) (157.7385, -11.8775) knots 0 0 0 1 2 2 2
  spline S123 degree 2 poles (157.7385, -11.8775) (158.1239, -11.9812) (159.2428, -12.248) (159.6133, -12.3591) knots 0 0 0 1 2 2 2
  spline S124 degree 2 poles (159.6133, -12.3591) (160.5544, -12.6481) (161.4287, -13.8115) (161.4287, -14.6637) knots 0 0 0 1 2 2 2
  spline S125 degree 2 poles (161.4287, -14.6637) (161.4287, -15.2046) (160.9915, -16.242) (160.5988, -16.6051) knots 0 0 0 1 2 2 2
  spline S126 degree 2 poles (160.5988, -16.6051) (160.1616, -17.0052) (159.0501, -17.435) (158.2128, -17.435) knots 0 0 0 1 2 2 2
  line L175 (168.1348, -9.2099) -> (163.8815, -9.2099)
  line L176 (163.8815, -9.2099) -> (163.8815, -11.7886)
  line L177 (163.8815, -11.7886) -> (167.957, -11.7886)
  line L178 (167.957, -11.7886) -> (167.957, -12.8704)
  line L179 (167.957, -12.8704) -> (163.8815, -12.8704)
  line L180 (163.8815, -12.8704) -> (163.8815, -17.272)
  line L181 (163.8815, -17.272) -> (162.6662, -17.272)
  line L182 (162.6662, -17.272) -> (162.6662, -8.128)
  line L183 (162.6662, -8.128) -> (168.1348, -8.128)
  line L184 (168.1348, -8.128) -> (168.1348, -9.2099)
  spline S127 degree 2 poles (175.6931, -9.1728) (176.2118, -9.7804) (176.7898, -11.5589) (176.7898, -12.7) knots 0 0 0 1 2 2 2
  spline S128 degree 2 poles (176.7898, -12.7) (176.7898, -13.8115) (176.2266, -15.6121) (175.6931, -16.2198) knots 0 0 0 1 2 2 2
  spline S129 degree 2 poles (175.6931, -16.2198) (175.1299, -16.857) (173.6405, -17.4647) (172.7439, -17.4647) knots 0 0 0 1 2 2 2
  spline S130 degree 2 poles (172.7439, -17.4647) (171.8176, -17.4647) (170.3356, -16.8348) (169.7947, -16.2198) knots 0 0 0 1 2 2 2
  spline S131 degree 2 poles (169.7947, -16.2198) (169.2686, -15.6121) (168.7054, -13.8263) (168.7054, -12.7) knots 0 0 0 1 2 2 2
  spline S132 degree 2 poles (168.7054, -12.7) (168.7054, -11.5514) (169.276, -9.8027) (169.8021, -9.1728) knots 0 0 0 1 2 2 2
  spline S133 degree 2 poles (169.8021, -9.1728) (170.3356, -8.5652) (171.825, -7.9353) (172.7439, -7.9353) knots 0 0 0 1 2 2 2
  spline S134 degree 2 poles (172.7439, -7.9353) (173.6775, -7.9353) (175.1744, -8.5874) (175.6931, -9.1728) knots 0 0 0 1 2 2 2
  spline S135 degree 2 poles (175.5227, -12.7) (175.5227, -11.796) (175.1299, -10.3955) (174.7742, -9.9361) knots 0 0 0 1 2 2 2
  spline S136 degree 2 poles (174.7742, -9.9361) (174.4111, -9.4618) (173.3886, -8.9876) (172.7513, -8.9876) knots 0 0 0 1 2 2 2
  spline S137 degree 2 poles (172.7513, -8.9876) (172.0918, -8.9876) (171.0989, -9.447) (170.7209, -9.9361) knots 0 0 0 1 2 2 2
  spline S138 degree 2 poles (170.7209, -9.9361) (170.3578, -10.4029) (169.9725, -11.8108) (169.9725, -12.7) knots 0 0 0 1 2 2 2
  spline S139 degree 2 poles (169.9725, -12.7) (169.9725, -14.5006) (171.4842, -16.4124) (172.7513, -16.4124) knots 0 0 0 1 2 2 2
  spline S140 degree 2 poles (172.7513, -16.4124) (174.0184, -16.4124) (175.5227, -14.5006) (175.5227, -12.7) knots 0 0 0 1 2 2 2
  line L185 (185.2002, -17.272) -> (183.6218, -17.272)
  line L186 (183.6218, -17.272) -> (180.7319, -13.6337)
  line L187 (180.7319, -13.6337) -> (179.3388, -13.6337)
  line L188 (179.3388, -13.6337) -> (179.3388, -17.272)
  line L189 (179.3388, -17.272) -> (178.1236, -17.272)
  line L190 (178.1236, -17.272) -> (178.1236, -8.128)
  line L191 (178.1236, -8.128) -> (180.48, -8.128)
  spline S141 degree 2 poles (180.48, -8.128) (181.2654, -8.128) (182.3251, -8.2984) (182.8067, -8.6097) knots 0 0 0 1 2 2 2
  spline S142 degree 2 poles (182.8067, -8.6097) (183.2884, -8.9209) (183.8441, -9.8916) (183.8441, -10.6104) knots 0 0 0 1 2 2 2
  spline S143 degree 2 poles (183.8441, -10.6104) (183.8441, -11.6107) (182.8215, -12.9668) (181.9472, -13.2928) knots 0 0 0 1 2 2 2
  line L192 (181.9472, -13.2928) -> (185.2002, -17.272)
  spline S144 degree 2 poles (182.577, -10.7067) (182.577, -10.3066) (182.2954, -9.6915) (181.999, -9.4914) knots 0 0 0 1 2 2 2
  spline S145 degree 2 poles (181.999, -9.4914) (181.7397, -9.321) (181.0505, -9.1802) (180.5467, -9.1802) knots 0 0 0 1 2 2 2
  line L193 (180.5467, -9.1802) -> (179.3388, -9.1802)
  line L194 (179.3388, -9.1802) -> (179.3388, -12.6185)
  line L195 (179.3388, -12.6185) -> (180.4059, -12.6185)
  spline S146 degree 2 poles (180.4059, -12.6185) (180.932, -12.6185) (181.7693, -12.4332) (182.0583, -12.1442) knots 0 0 0 1 2 2 2
  spline S147 degree 2 poles (182.0583, -12.1442) (182.3251, -11.8923) (182.577, -11.1809) (182.577, -10.7067) knots 0 0 0 1 2 2 2
  line L196 (193.7662, -17.272) -> (192.5509, -17.272)
  line L197 (192.5509, -17.272) -> (192.5509, -9.3951)
  line L198 (192.5509, -9.3951) -> (190.1649, -14.7526)
  line L199 (190.1649, -14.7526) -> (189.4239, -14.7526)
  line L200 (189.4239, -14.7526) -> (187.0601, -9.3951)
  line L201 (187.0601, -9.3951) -> (187.0601, -17.272)
  line L202 (187.0601, -17.272) -> (185.9264, -17.272)
  line L203 (185.9264, -17.272) -> (185.9264, -8.128)
  line L204 (185.9264, -8.128) -> (187.5862, -8.128)
  line L205 (187.5862, -8.128) -> (189.8685, -13.2187)
  line L206 (189.8685, -13.2187) -> (192.0767, -8.128)
  line L207 (192.0767, -8.128) -> (193.7662, -8.128)
  line L208 (193.7662, -8.128) -> (193.7662, -17.272)
  dimension "d18" = 203.2
  dimension "d19" = 10.16
  dimension "d20" = 0
  dimension "d21" = 25.4
  dimension "d22" = 7.62
  constraints: 2 other
  measures "d18" distance of L4.start L4.end